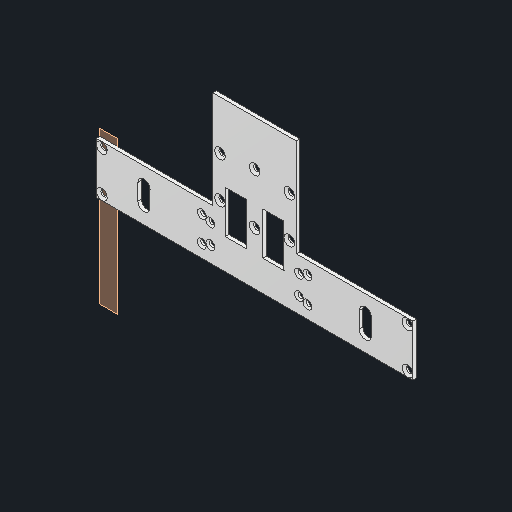
# Autodesk Inventor part: ceil
Saved by Autodesk Inventor 2023 (Build 270158000, 158)
## iProperties
Created: 2024-04-25
Part Number: ceil
Material: ABS Plastic
Document SubType Name: Modeling
Designer: szymo
Density: 1.06 g/cm^3
Appearance: Smooth - White
Mass: 14.1946 g
Surface Area: 153.158 cm^2
Volume: 13.3912 cm^3
Author: szymo
Autodesk Inventor part; units mm, degrees
ref_plane "YZ Plane" through (0, 0, 0) normal (1, 0, 0) x (0, 1, 0)
ref_plane "XZ Plane" through (0, 0, 0) normal (0, 1, 0) x (-1, 0, 0)
ref_plane "XY Plane" through (0, 0, 0) normal (0, 0, 1) x (1, 0, 0)
ref_plane "Work Plane1" through (0, 0, 0) normal (0, 0, 1) x (1, 0, 0)
ref_plane "Work Plane2" through (0, 0, 0) normal (0, 0, 1) x (1, 0, 0)
sketch "Sketch3" plane through (0, 0, 0) normal (0, 0, 1) x (1, 0, 0)
  circle A0 centre (3, -25.75) radius 2.3
  circle A1 centre (3, -3) radius 2.3
  circle A2 centre (3, -74.888889) radius 2.3
  line L0 (0, 0) -> (6, 0)
  line L1 (0, -77.888889) -> (0, 0)
  line L2 (0, -77.888889) -> (6, -77.888889)
  line L3 (6, -71.888889) -> (6, -77.888889)
  line L4 (6, -71.888889) -> (1.6, -71.888889)
  line L5 (1.6, -71.888889) -> (1.6, -56.788889)
  line L6 (1.6, -56.788889) -> (9.6, -56.788889)
  line L7 (9.6, -44.788889) -> (9.6, -56.788889)
  line L8 (3, -44.788889) -> (9.6, -44.788889)
  line L9 (3, -28.75) -> (3, -44.788889)
  line L10 (3, -28.75) -> (6, -28.75)
  line L11 (6, -28.75) -> (6, -22.75)
  line L12 (6, -22.75) -> (3, -22.75)
  line L13 (3, -6) -> (3, -22.75)
  line L14 (3, -6) -> (6, -6)
  line L15 (6, -6) -> (6, 0)
  circle A3 centre (5.6, -52.788889) radius 2.6
  circle A4 centre (175, -3) radius 2.3
  circle A5 centre (175, -25.75) radius 2.3
  line L16 (175, -28.75) -> (175, -41.888889)
  line L17 (168.4, -41.888889) -> (175, -41.888889)
  line L18 (168.4, -53.888889) -> (168.4, -41.888889)
  line L19 (175, -53.888889) -> (168.4, -53.888889)
  line L20 (175, -53.888889) -> (175, -71.888889)
  line L21 (172, -71.888889) -> (172, -77.888889)
  line L22 (178, -77.888889) -> (172, -77.888889)
  line L23 (178, -77.888889) -> (178, 0)
  line L24 (178, 0) -> (172, 0)
  line L25 (172, 0) -> (172, -6)
  line L26 (172, -6) -> (175, -6)
  line L27 (175, -6) -> (175, -22.75)
  line L28 (175, -22.75) -> (172, -22.75)
  line L29 (172, -22.75) -> (172, -28.75)
  line L30 (172, -28.75) -> (175, -28.75)
  circle A6 centre (175, -74.888889) radius 2.3
  circle A7 centre (172.4, -49.888889) radius 2.6
  circle A8 centre (89, 0.966057) radius 2.3
  circle A9 centre (89, 29.5) radius 2.3
  circle A10 centre (89, 15.55) radius 3.3
  circle A11 centre (89, -14.375) radius 3.3
  circle A12 centre (89, 41.2) radius 3.3
  line L31 (93.5, -27.75) -> (84.5, -27.75)
  line L32 (93.5, 55) -> (93.5, -27.75)
  line L33 (84.5, 55) -> (93.5, 55)
  line L34 (84.5, -27.75) -> (84.5, 55)
  line L35 (105.5, -27.75) -> (111.5, -27.75)
  line L36 (111.5, -24.910469) -> (111.5, -27.75)
  arc A13 (105.5, -24.910469) -> (111.5, -24.910469) centre (108.5, -23.95) ccw
  line L37 (105.5, -27.75) -> (105.5, -24.910469)
  arc A14 (111.5, -22.989531) -> (105.5, -22.989531) centre (108.5, -23.95) ccw
  line L38 (111.5, -5.585469) -> (111.5, -22.989531)
  arc A15 (105.5, -5.585469) -> (111.5, -5.585469) centre (108.5, -4.625) ccw
  line L39 (105.5, -22.989531) -> (105.5, -5.585469)
  circle A16 centre (108.484572, 4.5875) radius 2.3
  arc A17 (105.5, 12.839531) -> (111.5, 12.839531) centre (108.5, 13.8) ccw
  line L40 (105.5, -3.664531) -> (105.5, 12.839531)
  arc A18 (111.5, -3.664531) -> (105.5, -3.664531) centre (108.5, -4.625) ccw
  line L41 (111.5, 12.839531) -> (111.5, -3.664531)
  circle A19 centre (108.446201, 27.5) radius 2.3
  arc A20 (111.5, 14.760469) -> (105.5, 14.760469) centre (108.5, 13.8) ccw
  line L42 (111.5, 40.633122) -> (111.5, 14.760469)
  arc A21 (105.5, 40.133758) -> (111.5, 40.633122) centre (108.423077, 41.307692) ccw
  line L43 (105.5, 14.760469) -> (105.5, 40.133758)
  arc A22 (111.5, 41.982262) -> (105.5, 42.481626) centre (108.423077, 41.307692) ccw
  line L44 (111.5, 55) -> (111.5, 41.982262)
  line L45 (105.5, 55) -> (111.5, 55)
  line L46 (105.5, 42.481626) -> (105.5, 55)
  line L47 (111.5, 41.982262) -> (111.5, 55)
  line L48 (111.5, 41.982262) -> (112.5, 41.982262)
  line L49 (112.5, 41.982262) -> (112.5, 55)
  line L50 (111.5, 55) -> (112.5, 55)
  line L51 (111.5, 14.760469) -> (111.5, 40.633122)
  line L52 (111.5, 14.760469) -> (112.5, 14.760469)
  line L53 (112.5, 14.760469) -> (112.5, 40.633122)
  line L54 (111.5, 40.633122) -> (112.5, 40.633122)
  line L55 (111.5, -3.664531) -> (111.5, 12.839531)
  line L56 (111.5, -3.664531) -> (112.5, -3.664531)
  line L57 (112.5, -3.664531) -> (112.5, 12.839531)
  line L58 (111.5, 12.839531) -> (112.5, 12.839531)
  line L59 (66.5, 14.760469) -> (66.5, 40.633122)
  line L60 (66.5, 40.633122) -> (65.5, 40.633122)
  line L61 (65.5, 14.760469) -> (65.5, 40.633122)
  line L62 (66.5, 14.760469) -> (65.5, 14.760469)
  line L63 (66.5, 41.982262) -> (66.5, 55)
  line L64 (66.5, 55) -> (65.5, 55)
  line L65 (65.5, 41.982262) -> (65.5, 55)
  line L66 (66.5, 41.982262) -> (65.5, 41.982262)
  line L67 (66.5, -3.664531) -> (66.5, 12.839531)
  line L68 (66.5, 12.839531) -> (65.5, 12.839531)
  line L69 (65.5, -3.664531) -> (65.5, 12.839531)
  line L70 (66.5, -3.664531) -> (65.5, -3.664531)
  arc A23 (66.5, -5.585469) -> (72.5, -5.585469) centre (69.5, -4.625) ccw
  line L71 (66.5, -22.989531) -> (66.5, -5.585469)
  arc A24 (72.5, -22.989531) -> (66.5, -22.989531) centre (69.5, -23.95) ccw
  line L72 (72.5, -5.585469) -> (72.5, -22.989531)
  line L73 (66.5, -27.75) -> (72.5, -27.75)
  line L74 (72.5, -24.910469) -> (72.5, -27.75)
  arc A25 (66.5, -24.910469) -> (72.5, -24.910469) centre (69.5, -23.95) ccw
  line L75 (66.5, -27.75) -> (66.5, -24.910469)
  circle A26 centre (69.5, 4.5875) radius 2.3
  arc A27 (72.5, -3.664531) -> (66.5, -3.664531) centre (69.5, -4.625) ccw
  line L76 (72.5, 12.839531) -> (72.5, -3.664531)
  arc A28 (66.5, 12.839531) -> (72.5, 12.839531) centre (69.5, 13.8) ccw
  line L77 (66.5, -3.664531) -> (66.5, 12.839531)
  circle A29 centre (69.5, 27.5) radius 2.3
  arc A30 (66.5, 40.633122) -> (72.5, 40.133758) centre (69.576923, 41.307692) ccw
  line L78 (66.5, 14.760469) -> (66.5, 40.633122)
  arc A31 (72.5, 14.760469) -> (66.5, 14.760469) centre (69.5, 13.8) ccw
  line L79 (72.5, 40.133758) -> (72.5, 14.760469)
  arc A32 (72.5, 42.481626) -> (66.5, 41.982262) centre (69.576923, 41.307692) ccw
  line L80 (72.5, 55) -> (72.5, 42.481626)
  line L81 (66.5, 55) -> (72.5, 55)
  line L82 (66.5, 41.982262) -> (66.5, 55)
  circle A33 centre (59.3, -21.544506) radius 1.75
  circle A34 centre (59.3, -7.205494) radius 1.75
  line L83 (56.8, -28.75) -> (56.8, 0)
  line L84 (61.8, -28.75) -> (56.8, -28.75)
  line L85 (61.8, 0) -> (61.8, -28.75)
  line L86 (61.8, 0) -> (56.8, 0)
  circle A35 centre (64.05, -19.865715) radius 1.75
  circle A36 centre (64.05, -8.884285) radius 1.75
  line L87 (61.8, 0) -> (61.8, -28.75)
  line L88 (61.8, -28.75) -> (66.3, -28.75)
  line L89 (66.3, 0) -> (66.3, -28.75)
  line L90 (61.8, 0) -> (66.3, 0)
  circle A37 centre (113.95, -19.865715) radius 1.75
  circle A38 centre (113.95, -8.884285) radius 1.75
  line L91 (116.2, 0) -> (116.2, -28.75)
  line L92 (116.2, 0) -> (111.7, 0)
  line L93 (111.7, 0) -> (111.7, -28.75)
  line L94 (116.2, -28.75) -> (111.7, -28.75)
  circle A39 centre (118.7, -21.544506) radius 1.75
  circle A40 centre (118.7, -7.205494) radius 1.75
  line L95 (121.2, -28.75) -> (121.2, 0)
  line L96 (116.2, 0) -> (121.2, 0)
  line L97 (116.2, 0) -> (116.2, -28.75)
  line L98 (116.2, -28.75) -> (121.2, -28.75)
  line L99 (0, 0) -> (178, 0)
  line L100 (178, 0) -> (178, -28.75)
  line L101 (178, -28.75) -> (0, -28.75)
  line L102 (0, -28.75) -> (0, 0)
  line L103 (112.5, 0) -> (65.5, 0)
  line L104 (65.5, 0) -> (65.5, 55)
  line L105 (65.5, 55) -> (112.5, 55)
  line L106 (112.5, 55) -> (112.5, 0)
  line L107 (104.5, 11.432453) -> (104.5, -10.567547)
  line L108 (94.5, -10.567547) -> (94.5, 11.432453)
  line L109 (104.5, 11.432453) -> (73.5, 11.432453)
  line L110 (73.5, 11.432453) -> (73.5, -10.567547)
  line L111 (73.5, -10.567547) -> (104.5, -10.567547)
  line L112 (104.5, -10.567547) -> (104.5, 11.432453)
  line L113 (72.5, 12.432453) -> (105.5, 12.432453)
  line L114 (105.5, 12.432453) -> (105.5, -11.567547)
  line L115 (105.5, -11.567547) -> (72.5, -11.567547)
  line L116 (72.5, -11.567547) -> (72.5, 12.432453)
  line L117 (175, -71.888889) -> (172, -71.888889)
  line L118 (24.3, -9.775) -> (24.3, -18.975)
  line L119 (29.1, 0) -> (29.1, -28.75)
  spline S0 degree 3 poles (29.1, -9.775) (29.1, -9.463446) (29.036084, -9.135365) (28.780598, -8.535027) (28.5892, -8.26249) (28.160229, -7.849193) (27.899765, -7.673017) (27.321145, -7.43578) (27.002619, -7.375) (26.7, -7.375) (26.397381, -7.375) (26.078855, -7.43578) (25.500235, -7.673017) (25.239771, -7.849193) (24.8108, -8.26249) (24.619402, -8.535027) (24.363916, -9.135365) (24.3, -9.463446) (24.3, -9.775) knots -0.38002544 -0.38002544 -0.38002544 -0.38002544 -0.28079855 -0.28079855 -0.18157167 -0.18157167 -0.09078583 -0.09078583 0 0 0 0.09078583 0.09078583 0.18157167 0.18157167 0.28079855 0.28079855 0.38002544 0.38002544 0.38002544 0.38002544
  spline S1 degree 3 poles (24.3, -18.975) (24.3, -19.286554) (24.363916, -19.614635) (24.619402, -20.214973) (24.8108, -20.48751) (25.239771, -20.900807) (25.500235, -21.076983) (26.078855, -21.31422) (26.397381, -21.375) (27.002619, -21.375) (27.321145, -21.31422) (27.899765, -21.076983) (28.160229, -20.900807) (28.5892, -20.48751) (28.780598, -20.214973) (29.036084, -19.614635) (29.1, -19.286554) (29.1, -18.975) knots 0.36850475 0.36850475 0.36850475 0.36850475 0.46773163 0.46773163 0.56695852 0.56695852 0.65774435 0.65774435 0.74853018 0.74853018 0.83931602 0.83931602 0.93010185 0.93010185 1.02932873 1.02932873 1.12855562 1.12855562 1.12855562 1.12855562
  line L120 (153.7, -9.775) -> (153.7, -18.975)
  spline S2 degree 3 poles (153.7, -9.775) (153.7, -9.463446) (153.636084, -9.135365) (153.380598, -8.535027) (153.1892, -8.26249) (152.760229, -7.849193) (152.499765, -7.673017) (151.921145, -7.43578) (151.602619, -7.375) (151.3, -7.375) (150.997381, -7.375) (150.678855, -7.43578) (150.100235, -7.673017) (149.839771, -7.849193) (149.4108, -8.26249) (149.219402, -8.535027) (148.963916, -9.135365) (148.9, -9.463446) (148.9, -9.775) knots -0.38002544 -0.38002544 -0.38002544 -0.38002544 -0.28079855 -0.28079855 -0.18157167 -0.18157167 -0.09078583 -0.09078583 0 0 0 0.09078583 0.09078583 0.18157167 0.18157167 0.28079855 0.28079855 0.38002544 0.38002544 0.38002544 0.38002544
  line L121 (148.9, 0) -> (148.9, -28.75)
  spline S3 degree 3 poles (148.9, -18.975) (148.9, -19.286554) (148.963916, -19.614635) (149.219402, -20.214973) (149.4108, -20.48751) (149.839771, -20.900807) (150.100235, -21.076983) (150.678855, -21.31422) (150.997381, -21.375) (151.602619, -21.375) (151.921145, -21.31422) (152.499765, -21.076983) (152.760229, -20.900807) (153.1892, -20.48751) (153.380598, -20.214973) (153.636084, -19.614635) (153.7, -19.286554) (153.7, -18.975) knots 0.36850475 0.36850475 0.36850475 0.36850475 0.46773163 0.46773163 0.56695852 0.56695852 0.65774435 0.65774435 0.74853018 0.74853018 0.83931602 0.83931602 0.93010185 0.93010185 1.02932873 1.02932873 1.12855562 1.12855562 1.12855562 1.12855562
  line L122 (23.3, -9.775) -> (23.3, -18.975)
  line L123 (30.1, 0) -> (30.1, -28.75)
  line L124 (154.7, -9.775) -> (154.7, -18.975)
  line L125 (147.9, 0) -> (147.9, -28.75)
  spline S4 degree 5 poles (30.1, -9.775) (30.100329, -9.424272) (30.052087, -9.074692) (29.965589, -8.730751) (29.697027, -8.078799) (29.275424, -7.514739) (29.030017, -7.260888) (28.461662, -6.814655) (27.798444, -6.523394) (27.437569, -6.42799) (26.7, -6.321903) (25.962431, -6.42799) (25.601556, -6.523394) (24.938338, -6.814655) (24.369983, -7.260888) (24.124576, -7.514739) (23.702973, -8.078799) (23.434411, -8.730751) (23.347913, -9.074692) (23.299671, -9.424272) (23.3, -9.775) knots 0 0 0 0 0 0 0.16408941 0.16408941 0.16408941 0.32727987 0.32727987 0.32727987 0.5 0.5 0.5 0.67272013 0.67272013 0.67272013 0.83591059 0.83591059 0.83591059 1 1 1 1 1 1
  spline S5 degree 5 poles (23.3, -18.975) (23.299671, -19.325728) (23.347913, -19.675308) (23.434411, -20.019249) (23.702973, -20.671201) (24.124576, -21.235261) (24.369983, -21.489112) (24.938338, -21.935345) (25.601556, -22.226606) (25.962431, -22.32201) (26.7, -22.428097) (27.437569, -22.32201) (27.798444, -22.226606) (28.461662, -21.935345) (29.030017, -21.489112) (29.275424, -21.235261) (29.697027, -20.671201) (29.965589, -20.019249) (30.052087, -19.675308) (30.100329, -19.325728) (30.1, -18.975) knots 0 0 0 0 0 0 0.16408941 0.16408941 0.16408941 0.32727987 0.32727987 0.32727987 0.5 0.5 0.5 0.67272013 0.67272013 0.67272013 0.83591059 0.83591059 0.83591059 1 1 1 1 1 1
  spline S6 degree 5 poles (147.9, -9.775) (147.899671, -9.424272) (147.947913, -9.074692) (148.034411, -8.730751) (148.302973, -8.078799) (148.724576, -7.514739) (148.969983, -7.260888) (149.538338, -6.814655) (150.201556, -6.523394) (150.562431, -6.42799) (151.3, -6.321903) (152.037569, -6.42799) (152.398444, -6.523394) (153.061662, -6.814655) (153.630017, -7.260888) (153.875424, -7.514739) (154.297027, -8.078799) (154.565589, -8.730751) (154.652087, -9.074692) (154.700329, -9.424272) (154.7, -9.775) knots 0 0 0 0 0 0 0.16408941 0.16408941 0.16408941 0.32727987 0.32727987 0.32727987 0.5 0.5 0.5 0.67272013 0.67272013 0.67272013 0.83591059 0.83591059 0.83591059 1 1 1 1 1 1
  spline S7 degree 5 poles (154.7, -18.975) (154.700329, -19.325728) (154.652087, -19.675308) (154.565589, -20.019249) (154.297027, -20.671201) (153.875424, -21.235261) (153.630017, -21.489112) (153.061662, -21.935345) (152.398444, -22.226606) (152.037569, -22.32201) (151.3, -22.428097) (150.562431, -22.32201) (150.201556, -22.226606) (149.538338, -21.935345) (148.969983, -21.489112) (148.724576, -21.235261) (148.302973, -20.671201) (148.034411, -20.019249) (147.947913, -19.675308) (147.899671, -19.325728) (147.9, -18.975) knots 0 0 0 0 0 0 0.16408941 0.16408941 0.16408941 0.32727987 0.32727987 0.32727987 0.5 0.5 0.5 0.67272013 0.67272013 0.67272013 0.83591059 0.83591059 0.83591059 1 1 1 1 1 1
  point P0 (112.5, 0)
  point P1 (65.5, 0)
  point P2 (0, -28.75)
  point P3 (172, 0)
  point P4 (93.5, 12.432453)
  point P5 (105.5, -5.585469)
  point P6 (93.5, -11.567547)
  point P7 (84.5, -11.567547)
  point P8 (72.5, -5.585469)
  point P9 (84.5, 12.432453)
  point P10 (30.1, -9.775)
  point P11 (30.1, -18.975)
  point P12 (147.9, -18.975)
  point P13 (147.9, -9.775)
  dimension "d34" = 1
  dimension "d36" = 1
  dimension "d29" = 1
  dimension "d30" = 1
  dimension "d31" = 1
  dimension "d35" = 1
  dimension "d37" = 1
  constraints: 40 end point, 14 parallel, 5 point on line, 4 perpendicular, 3 horizontal, 15 other
  measures "d29" distance between parallel lines of L107 L40
  measures "d30" distance between parallel lines of L76 L110
  measures "d31" distance between parallel lines of L109 L113
  measures "d35" distance between parallel lines of L119 L123
  measures "d37" distance between parallel lines of L121 L125
sketch "Sketch3 outline for Extrusion2" plane through (0, 0, 0) normal (0, 0, 1) x (1, 0, 0)
  line L0 (112.5, 0) -> (112.5, 12.839531)
  line L1 (116.2, 0) -> (112.5, 0)
  line L2 (112.5, 12.839531) -> (112.5, 14.760469)
  line L3 (121.2, 0) -> (116.2, 0)
  line L4 (112.5, 14.760469) -> (112.5, 40.633122)
  line L5 (172, 0) -> (121.2, 0)
  line L6 (112.5, 40.633122) -> (112.5, 41.982262)
  line L7 (178, 0) -> (172, 0)
  line L8 (112.5, 41.982262) -> (112.5, 55)
  line L9 (178, -28.75) -> (178, 0)
  line L10 (112.5, 55) -> (111.5, 55)
  line L11 (175, -28.75) -> (178, -28.75)
  line L12 (111.5, 55) -> (105.5, 55)
  line L13 (172, -28.75) -> (175, -28.75)
  line L14 (105.5, 55) -> (93.5, 55)
  line L15 (121.2, -28.75) -> (172, -28.75)
  line L16 (93.5, 55) -> (84.5, 55)
  line L17 (116.2, -28.75) -> (121.2, -28.75)
  line L18 (84.5, 55) -> (72.5, 55)
  line L19 (111.7, -28.75) -> (116.2, -28.75)
  line L20 (72.5, 55) -> (66.5, 55)
  line L21 (66.3, -28.75) -> (111.7, -28.75)
  line L22 (66.5, 55) -> (65.5, 55)
  line L23 (61.8, -28.75) -> (66.3, -28.75)
  line L24 (65.5, 55) -> (65.5, 41.982262)
  line L25 (56.8, -28.75) -> (61.8, -28.75)
  line L26 (65.5, 41.982262) -> (65.5, 40.633122)
  line L27 (6, -28.75) -> (56.8, -28.75)
  line L28 (65.5, 40.633122) -> (65.5, 14.760469)
  line L29 (3, -28.75) -> (6, -28.75)
  line L30 (65.5, 14.760469) -> (65.5, 12.839531)
  line L31 (0, -28.75) -> (3, -28.75)
  line L32 (65.5, 12.839531) -> (65.5, 0)
  line L33 (0, 0) -> (0, -28.75)
  line L34 (65.5, 0) -> (61.8, 0)
  line L35 (6, 0) -> (0, 0)
  line L36 (61.8, 0) -> (56.8, 0)
  line L37 (56.8, 0) -> (6, 0)
  spline S0 degree 5 poles (23.3, -18.975) (23.299671, -19.325728) (23.347913, -19.675308) (23.434411, -20.019249) (23.702973, -20.671201) (24.124576, -21.235261) (24.369983, -21.489112) (24.938338, -21.935345) (25.601556, -22.226606) (25.962431, -22.32201) (26.7, -22.428097) (27.437569, -22.32201) (27.798444, -22.226606) (28.461662, -21.935345) (29.030017, -21.489112) (29.275424, -21.235261) (29.697027, -20.671201) (29.965589, -20.019249) (30.052087, -19.675308) (30.100329, -19.325728) (30.1, -18.975) knots 0 0 0 0 0 0 0.16408941 0.16408941 0.16408941 0.32727987 0.32727987 0.32727987 0.5 0.5 0.5 0.67272013 0.67272013 0.67272013 0.83591059 0.83591059 0.83591059 1 1 1 1 1 1
  line L38 (30.1, -9.775) -> (30.1, -18.975)
  spline S1 degree 5 poles (30.1, -9.775) (30.100329, -9.424272) (30.052087, -9.074692) (29.965589, -8.730751) (29.697027, -8.078799) (29.275424, -7.514739) (29.030017, -7.260888) (28.461662, -6.814655) (27.798444, -6.523394) (27.437569, -6.42799) (26.7, -6.321903) (25.962431, -6.42799) (25.601556, -6.523394) (24.938338, -6.814655) (24.369983, -7.260888) (24.124576, -7.514739) (23.702973, -8.078799) (23.434411, -8.730751) (23.347913, -9.074692) (23.299671, -9.424272) (23.3, -9.775) knots 0 0 0 0 0 0 0.16408941 0.16408941 0.16408941 0.32727987 0.32727987 0.32727987 0.5 0.5 0.5 0.67272013 0.67272013 0.67272013 0.83591059 0.83591059 0.83591059 1 1 1 1 1 1
  line L39 (23.3, -18.975) -> (23.3, -9.775)
  line L40 (147.9, -18.975) -> (147.9, -9.775)
  spline S2 degree 5 poles (154.7, -18.975) (154.700329, -19.325728) (154.652087, -19.675308) (154.565589, -20.019249) (154.297027, -20.671201) (153.875424, -21.235261) (153.630017, -21.489112) (153.061662, -21.935345) (152.398444, -22.226606) (152.037569, -22.32201) (151.3, -22.428097) (150.562431, -22.32201) (150.201556, -22.226606) (149.538338, -21.935345) (148.969983, -21.489112) (148.724576, -21.235261) (148.302973, -20.671201) (148.034411, -20.019249) (147.947913, -19.675308) (147.899671, -19.325728) (147.9, -18.975) knots 0 0 0 0 0 0 0.16408941 0.16408941 0.16408941 0.32727987 0.32727987 0.32727987 0.5 0.5 0.5 0.67272013 0.67272013 0.67272013 0.83591059 0.83591059 0.83591059 1 1 1 1 1 1
  line L41 (154.7, -9.775) -> (154.7, -18.975)
  spline S3 degree 5 poles (147.9, -9.775) (147.899671, -9.424272) (147.947913, -9.074692) (148.034411, -8.730751) (148.302973, -8.078799) (148.724576, -7.514739) (148.969983, -7.260888) (149.538338, -6.814655) (150.201556, -6.523394) (150.562431, -6.42799) (151.3, -6.321903) (152.037569, -6.42799) (152.398444, -6.523394) (153.061662, -6.814655) (153.630017, -7.260888) (153.875424, -7.514739) (154.297027, -8.078799) (154.565589, -8.730751) (154.652087, -9.074692) (154.700329, -9.424272) (154.7, -9.775) knots 0 0 0 0 0 0 0.16408941 0.16408941 0.16408941 0.32727987 0.32727987 0.32727987 0.5 0.5 0.5 0.67272013 0.67272013 0.67272013 0.83591059 0.83591059 0.83591059 1 1 1 1 1 1
  line L42 (84.5, 12.432453) -> (84.5, -11.567547)
  line L43 (72.5, 12.432453) -> (84.5, 12.432453)
  line L44 (72.5, -3.664531) -> (72.5, 12.432453)
  line L45 (72.5, -5.585469) -> (72.5, -3.664531)
  line L46 (72.5, -11.567547) -> (72.5, -5.585469)
  line L47 (84.5, -11.567547) -> (72.5, -11.567547)
  line L48 (93.5, -11.567547) -> (93.5, 12.432453)
  line L49 (105.5, -11.567547) -> (93.5, -11.567547)
  line L50 (105.5, -5.585469) -> (105.5, -11.567547)
  line L51 (105.5, -3.664531) -> (105.5, -5.585469)
  line L52 (105.5, 12.432453) -> (105.5, -3.664531)
  line L53 (93.5, 12.432453) -> (105.5, 12.432453)
extrude "Extrusion2" add sketch "Sketch3 outline for Extrusion2" along normal blind 2
sketch "Sketch4" plane through (0, 0, 2) normal (0, 0, 1) x (1, 0, 0)
  circle A0 centre (69.5, 27.5) radius 2.3
  circle A1 centre (69.5, 4.5875) radius 2.3
  circle A2 centre (89, 0.966057) radius 2
  circle A3 centre (89, 29.5) radius 2.3
  circle A4 centre (108.446201, 27.5) radius 2.3
  circle A5 centre (108.484572, 4.5875) radius 2.3
  circle A6 centre (64.05, -8.884285) radius 1.75
  circle A7 centre (59.3, -7.205494) radius 1.75
  circle A8 centre (59.3, -21.544506) radius 1.75
  circle A9 centre (64.05, -19.865715) radius 1.75
  circle A10 centre (118.7, -21.544506) radius 1.75
  circle A11 centre (113.95, -19.865715) radius 1.75
  circle A12 centre (113.95, -8.884285) radius 1.75
  circle A13 centre (118.7, -7.205494) radius 1.75
  circle A14 centre (3, -25.75) radius 2.3
  circle A15 centre (3, -3) radius 2.3
  circle A16 centre (175, -25.75) radius 2.3
  circle A17 centre (175, -3) radius 2.3
  point P0 (0, 0)
  constraints: 18 coincident
hole "Hole2" at (3, -3, 2) at (3, -25.75, 2) at (175, -3, 2) at (175, -25.75, 2) at (108.484572, 4.5875, 2) at (89, 0.966057, 2) at (69.5, 4.5875, 2) at (69.5, 27.5, 2) at (89, 29.5, 2) at (108.446201, 27.5, 2) direction (0, 0, -1) diameter 3.6 end through all countersink diameter 6 countersink angle 90 clearance for "Countersunk Flat Head Screw ISO 2009/7046" size "M3" standard "ISO"
sketch "Sketch5" plane through (0, 0, 2) normal (0, 0, 1) x (1, 0, 0)
  circle A0 centre (64.05, -19.865715) radius 1.75
  circle A1 centre (59.3, -21.544506) radius 1.75
  circle A2 centre (59.3, -7.205494) radius 1.75
  circle A3 centre (64.05, -8.884285) radius 1.75
  circle A4 centre (113.95, -8.884285) radius 1.75
  circle A5 centre (118.7, -7.205494) radius 1.75
  circle A6 centre (118.7, -21.544506) radius 1.75
  circle A7 centre (113.95, -19.865715) radius 1.75
  point P0 (0, 0)
  constraints: 8 coincident
hole "Hole3" at (59.3, -7.205494, 2) at (64.05, -8.884285, 2) at (64.05, -19.865715, 2) at (59.3, -21.544506, 2) at (113.95, -8.884285, 2) at (118.7, -7.205494, 2) at (118.7, -21.544506, 2) at (113.95, -19.865715, 2) direction (0, 0, -1) diameter 3.1 end through all countersink diameter 5 countersink angle 90 clearance for "Countersunk Flat Head Screw ISO 2009/7046" size "M2.5" standard "ISO"
equation "\"d30\" = d29"
body "Solid2"
